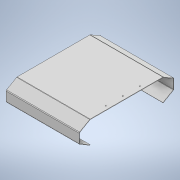
# Autodesk Inventor part: topBody
Saved by Autodesk Inventor 2020.3 (Build 243373000, 373)
## iProperties
Created: 2022-07-13
Part Number: topBody
Material: Generic
Document SubType Name: Sheet Metal
Designer: 0x6f736f646f
Density: 1 g/cm^3
Sheet Metal Rule: Default_mm
Appearance: Default
Author: 0x6f736f646f
Autodesk Inventor part; units mm, degrees
ref_plane "YZ Plane" through (0, 0, 0) normal (1, 0, 0) x (0, 1, 0)
ref_plane "XZ Plane" through (0, 0, 0) normal (0, 1, 0) x (-1, 0, 0)
ref_plane "XY Plane" through (0, 0, 0) normal (0, 0, 1) x (1, 0, 0)
sketch "Sketch1" plane through (0, 0, 0) normal (0, 1, 0) x (-1, 0, 0)
  line L0 (150, 290) -> (-150, 290)
  line L1 (-150, 290) -> (-150, -290)
  line L2 (-150, -290) -> (150, -290)
  line L3 (150, -290) -> (150, 290)
  line L4 (0, -406) -> (0, 406) projected
  line L5 (210, 0) -> (-210, 0) projected
  line L6 (150, 240) -> (-150, 240)
  line L7 (150, 200) -> (-150, 200)
  line L8 (150, 0) -> (-150, 0)
  line L9 (150, -240) -> (-150, -240)
  line L10 (150, -200) -> (-150, -200)
  line L11 (150, 290) -> (110, 240)
  line L12 (110, 200) -> (150, 150)
  line L13 (110, 200) -> (110, 240)
  line L14 (150, -290) -> (110, -240)
  line L15 (110, -200) -> (150, -150)
  line L16 (110, -200) -> (110, -240)
  line L17 (-150, 290) -> (-110, 240)
  line L18 (-110, 200) -> (-150, 150)
  line L19 (-110, 200) -> (-110, 240)
  line L20 (-150, -290) -> (-110, -240)
  line L21 (-110, -200) -> (-150, -150)
  line L22 (-110, -200) -> (-110, -240)
  line L23 (150, 150) -> (-150, 150)
  line L24 (150, -150) -> (-150, -150)
  circle A0 centre (-95, 220) radius 2
  circle A1 centre (-93.7861, 175) radius 2
  circle A2 centre (-135, 70) radius 2
  circle A3 centre (-135, 0) radius 2
  circle A4 centre (-135, -70) radius 2
  circle A5 centre (-108.2515, -178.1739) radius 2
  circle A6 centre (-95, -220) radius 2
  point P0 (0, 0)
  point P1 (0, -290)
  dimension "d0" = 300
  dimension "d1" = 50
  dimension "d3" = 40
  dimension "d50" = 40
  dimension "d51" = 300
  dimension "d52" = 50
  dimension "d89" = 4
  dimension "d90" = 4
  dimension "d91" = 4
  dimension "d92" = 4
  dimension "d93" = 4
  dimension "d94" = 4
  dimension "d95" = 4
  dimension "d96" = 15
  dimension "d97" = 20
  dimension "d98" = 15
  dimension "d99" = 15
  dimension "d100" = 70
  dimension "d101" = 15
  dimension "d102" = 0
  dimension "d103" = 70
  dimension "d104" = 15
  dimension "d105" = 15
  dimension "d106" = 20
  constraints: 46 end point, 14 symmetric about line, 10 point on line, 7 centre point, 3 midpoint, 3 parallel, 2 perpendicular, 1 horizontal, 1 vertical
  measures "d0" distance between parallel lines of L1 L3
  measures "d1" distance between parallel lines of L0 L6
  measures "d3" distance between parallel lines of L6 L7
  measures "d50" distance between parallel lines of L13 L3
  measures "d51" distance between parallel lines of L24 L23
  measures "d52" distance between parallel lines of L23 L7
  measures "d89" diameter of A0
  measures "d90" diameter of A1
  measures "d91" diameter of A2
  measures "d92" diameter of A3
  measures "d93" diameter of A4
  measures "d94" diameter of A5
  measures "d95" diameter of A6
  measures "d96" distance from line of L22 A6.centre
  measures "d97" distance from line of L9 A6.centre
  measures "d98" distance from line of L21 A5.centre
  measures "d99" distance from line of L1 A4.centre
  measures "d100" distance from line of L5 A4.centre
  measures "d101" distance from line of L1 A3.centre
  measures "d102" distance from line of L5 A3.centre
  measures "d103" distance from line of L5 A2.centre
  measures "d104" distance from line of L1 A2.centre
  measures "d105" distance from line of L19 A0.centre
  measures "d106" distance from line of L7 A0.centre
extrude "Plate1" add sketch "Sketch1" along normal blind 2 contours L11 L6 L4 L0 | L3 L6 L11 | L4 L6 L17 L0 | L3 L7 L13 L6 | L13 L7 L4 L6 | L17 L6 L1 | L4 L7 L19 L6 | L3 L12 L7 | L12 L23 L4 L7 | L6 L19 L7 L1 | L4 L23 L18 L7 | L3 L5 L4 L23 | L7 L18 L1 | L4 L5 A3 L1 L23 | L3 L24 L4 L5 | L4 L24 L1 L5 A3 | L3 L10 L15 | L15 L10 L4 L24 | L4 L10 L21 L24 | A3 L5 | L5 A3 | L3 L9 L16 L10 | L16 L9 L4 L10 | L21 L10 L1 | L4 L9 L22 L10 | L3 L14 L9 | L14 L2 L4 L9 | L10 L22 L9 L1 | L4 L2 L20 L9 | L9 L20 L1 | A0 | A1 | A2 | A4 | A5 | A6
fold "Fold7" angle 60 bend radius 2 thickness 2 k factor 0.44 line from (-150, 0, 240) to (150, 0, 240) line at bend centre moving side (0, 0, 1) folds toward (0, -1, 0)
fold "Fold8" angle 60 bend radius 2 thickness 2 k factor 0.44 line from (-150, 0, 200) to (150, 0, 200) line at bend centre moving side (0, 0, 1) folds toward (0, -1, 0)
fold "Fold9" angle 30 bend radius 2 thickness 2 k factor 0.44 line from (-150, 0, 150) to (150, 0, 150) line at bend centre moving side (0, 0, 1) folds toward (0, -1, 0)
fold "Fold10" angle 60 bend radius 2 thickness 2 k factor 0.44 line from (-150, 0, -240) to (150, 0, -240) line at bend centre moving side (0, 0, -1) folds toward (0, -1, 0)
fold "Fold11" angle 60 bend radius 2 thickness 2 k factor 0.44 line from (-150, 0, -200) to (150, 0, -200) line at bend centre moving side (0, 0, -1) folds toward (0, -1, 0)
fold "Fold12" angle 30 bend radius 2 thickness 2 k factor 0.44 line from (-150, 0, -150) to (150, 0, -150) line at bend centre moving side (0, 0, -1) folds toward (0, -1, 0)
hole "Hole1" at (135, 0, 70) direction (0, 1, 0) diameter 4 end through all
hole "Hole2" at (135, 0, 0) direction (0, 1, 0) diameter 4 end through all
hole "Hole3" at (135, 0, -70) direction (0, 1, 0) diameter 4 end through all
equation "\"d5\" = Thickness"
equation "\"d53\" = BendReliefWidth"
equation "\"d54\" = BendReliefDepth"
equation "\"d55\" = MinimumRemnant"
equation "\"d56\" = TransitionRadius"
equation "\"d58\" = BendRadius"
equation "\"d59\" = BendReliefWidth"
equation "\"d60\" = BendReliefDepth"
equation "\"d61\" = MinimumRemnant"
equation "\"d62\" = TransitionRadius"
equation "\"d64\" = BendRadius"
equation "\"d65\" = BendReliefWidth"
equation "\"d66\" = BendReliefDepth"
equation "\"d67\" = MinimumRemnant"
equation "\"d68\" = TransitionRadius"
equation "\"d70\" = BendRadius"
equation "\"d71\" = BendReliefWidth"
equation "\"d72\" = BendReliefDepth"
equation "\"d73\" = MinimumRemnant"
equation "\"d74\" = TransitionRadius"
equation "\"d76\" = BendRadius"
equation "\"d77\" = BendReliefWidth"
equation "\"d78\" = BendReliefDepth"
equation "\"d79\" = MinimumRemnant"
equation "\"d80\" = TransitionRadius"
equation "\"d82\" = BendRadius"
equation "\"d83\" = BendReliefWidth"
equation "\"d84\" = BendReliefDepth"
equation "\"d85\" = MinimumRemnant"
equation "\"d86\" = TransitionRadius"
equation "\"d88\" = BendRadius"
equation "\"d112\" = Thickness"
equation "\"d119\" = Thickness"
equation "\"d126\" = Thickness"
equation "\"BendRadius\" = Thickness"
equation "\"BendReliefWidth\" = Thickness"
equation "\"BendReliefDepth\" = 0.5 * Thickness"
equation "\"CornerReliefSize\" = 4 * Thickness"
equation "\"MinimumRemnant\" = 2 * Thickness"
equation "\"TransitionRadius\" = BendRadius"
equation "\"JacobiRadiusSize\" = BendRadius"
equation "\"GapSize\" = Thickness"
equation "\"Thickness\" = 2"
body "Solid1"
